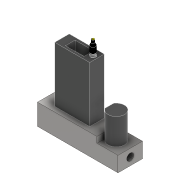
# Autodesk Inventor part: alicat_flujo
Saved by Autodesk Inventor 2022 (Build 260153000, 153)
## iProperties
Created: 2022-11-15
Part Number: alicat_flujo
Material: Generic
Document SubType Name: Modeling
Designer: ferna
Density: 1 g/cm^3
Appearance: Default
Author: ferna
Autodesk Inventor part; units mm, degrees
ref_plane "YZ Plane" through (0, 0, 0) normal (1, 0, 0) x (0, 1, 0)
ref_plane "XZ Plane" through (0, 0, 0) normal (0, 1, 0) x (-1, 0, 0)
sketch "Sketch1" plane through (0, 0, 0) normal (0, 1, 0) x (-1, 0, 0)
  line L0 (0, 0) -> (138, 0)
  line L1 (138, 0) -> (138, -42)
  line L2 (138, -42) -> (0, -42)
  line L3 (0, -42) -> (0, 0)
  dimension "d0" = 138
  dimension "d1" = 42
  constraints: 8 end point, 2 parallel, 1 horizontal, 1 perpendicular
  measures "d0" distance of L1.end L2.end
  measures "d1" distance of L0.end L1.end
extrude "Extrusion1" add sketch "Sketch1" along normal blind 26
sketch "Sketch2" plane through (0, 26, 0) normal (0, 1, 0) x (1, 0, 0)
  line L0 (-138, 42) -> (-138, 0) projected
  line L1 (0, 42) -> (-138, 42) projected
  line L2 (-138, 0) -> (-36, 0)
  line L3 (-36, 0) -> (-36, 42)
  line L4 (-36, 42) -> (-138, 42)
  line L5 (-138, 42) -> (-138, 0)
  point P0 (0, 0)
  dimension "d4" = 102
  constraints: 8 end point, 2 parallel, 1 horizontal, 1 perpendicular, 1 point on line
  measures "d4" distance of L4.end L3.end
extrude "Extrusion2" add sketch "Sketch2" along normal blind 10
sketch "Sketch3" plane through (0, 26, 0) normal (0, 1, 0) x (1, 0, 0)
  line L0 (-36, 0) -> (-36, 42) projected
  line L1 (-36, 21) -> (-24, 21)
  arc A0 (-36, 13.7889) -> (-36, 28.2111) centre (-24, 21) ccw
  line L2 (-36, 13.7889) -> (-36, 28.2111)
  point P0 (0, 0)
  dimension "d7" = 12
  dimension "d8" = 14
  constraints: 4 end point, 2 point on circle, 1 centre point, 1 coincident, 1 collinear, 1 horizontal, 1 midpoint, 1 point on line
  measures "d7" distance of L1.start L1.end
  measures "d8" radius of A0
extrude "Extrusion3" add sketch "Sketch3" along normal blind 45
sketch "Sketch4" plane through (0, 36, 0) normal (0, 1, 0) x (1, 0, 0)
  line L0 (-138, 42) -> (-138, 0) projected
  line L1 (-138, 0) -> (-87, 0)
  line L2 (-138, 0) -> (-36, 0) projected
  line L3 (-87, 0) -> (-87, 21)
  line L4 (-36, 42) -> (-138, 42) projected
  line L5 (-57, 8.5) -> (-117, 8.5)
  line L6 (-117, 8.5) -> (-117, 33.5)
  line L7 (-117, 33.5) -> (-57, 33.5)
  line L8 (-57, 33.5) -> (-57, 8.5)
  line L9 (-57, 8.5) -> (-117, 33.5) construction
  line L10 (-117, 8.5) -> (-57, 33.5) construction
  point P0 (0, 0)
  dimension "d11" = 21
  dimension "d12" = 60
  dimension "d13" = 25
  constraints: 16 end point, 3 midpoint, 2 parallel, 2 perpendicular, 1 horizontal
  measures "d11" distance of L1.end L3.end
  measures "d12" distance of L6.end L7.end
  measures "d13" distance of L5.end L6.end
extrude "Extrusion4" add sketch "Sketch4" along normal blind 95
sketch "Sketch6" plane through (-138, 0, 0) normal (0, 0, 1) x (1, 0, 0)
  line L0 (138, 26) -> (102, 26) projected
  line L1 (102, 26) -> (138, 26)
  line L2 (138, 26) -> (138, 79.7239)
  line L3 (138, 79.7239) -> (98.9473, 78.614)
  line L4 (102, 26) -> (102, 36) projected
  line L5 (98.9473, 78.614) -> (102, 36)
  line L6 (102, 36) -> (102, 26)
  point P0 (138, 0)
  constraints: 10 end point, 2 collinear, 1 perpendicular
split body "Split1" sketch "Sketch6" result two bodies curves L2 L3 L5 L6 L1 first body at (-23.4126, 56, -34.4872)
sketch "Sketch7" plane through (-138, 0, 0) normal (0, 0, 1) x (1, 0, 0)
  line L0 (81, 36) -> (21, 36) projected
  line L1 (81, 36) -> (81, 131) projected
  line L2 (21, 131) -> (81, 131) projected
  line L3 (21, 36) -> (21, 131) projected
  point P0 (138, 0)
split body "Split2" sketch "Sketch7" result two bodies bodies 3 curves L1 L2 L3 L0 first body at (-97, 67.6667, -9)
sketch "Sketch8" plane through (0, 0, 0) normal (1, 0, 0) x (0, 0, -1)
  line L0 (0, 0) -> (42, 0) projected
  line L1 (21, 0) -> (21, 13)
  circle A0 centre (21, 13) radius 6
  dimension "d16" = 13
  dimension "d17" = 12
  constraints: 2 end point, 1 centre point, 1 coincident, 1 midpoint, 1 vertical
  measures "d16" distance of L1.start L1.end
  measures "d17" diameter of A0
extrude "Extrusion5" cut sketch "Sketch8" against normal blind 20 bodies 5
sketch "Sketch9" plane through (-138, 0, -42) normal (-1, 0, 0) x (0, 0, 1)
  circle A0 centre (21, 13) radius 6 projected
  point P0 (42, 0)
extrude "Extrusion6" cut sketch "Sketch9" against normal blind 20 bodies 5
thread "Thread1" size "M12x1.75" class "6H" standard "ANSI Metric M Profile" full length
sketch "Sketch12" plane through (-57, 131, -33.5) normal (0, 0, -1) x (-1, 0, 0)
  line L0 (0.306, -7.7857) -> (59.5727, -7.7857) construction
  line L1 (59.5727, -7.7857) -> (59.5727, -94.7807) construction
  line L2 (59.5727, -94.7807) -> (0.306, -94.7807) construction
  line L3 (0.306, -94.7807) -> (0.306, -7.7857) construction
  point P0 (-57, -131)
  constraints: 2 other
decal "Decal2"
sketch "Sketch13" plane through (0, 131, 0) normal (0, 1, 0) x (1, 0, 0)
  line L0 (-117, 33.5) -> (-117, 8.5) projected
  line L1 (-117, 21) -> (-87, 21)
  line L2 (-102.9, 29.325) -> (-71.1, 29.325)
  line L3 (-71.1, 29.325) -> (-71.1, 12.675)
  line L4 (-71.1, 12.675) -> (-102.9, 12.675)
  line L5 (-102.9, 12.675) -> (-102.9, 29.325)
  line L6 (-102.9, 29.325) -> (-71.1, 12.675) construction
  line L7 (-71.1, 29.325) -> (-102.9, 12.675) construction
  point P0 (0, 0)
  dimension "d38" = 30
  dimension "d39" = 31.8
  dimension "d40" = 16.65
  constraints: 14 end point, 3 midpoint, 2 horizontal, 2 parallel, 1 perpendicular
  measures "d38" distance of L1.start L1.end
  measures "d39" distance of L3.end L4.end
  measures "d40" distance of L2.end L3.end
extrude "Extrusion7" cut sketch "Sketch13" against normal blind 16.2 bodies 4
sketch "Sketch14" plane through (0, 131, 0) normal (0, 1, 0) x (1, 0, 0)
  line L0 (-71.1, 29.325) -> (-71.1, 12.675) projected
  line L1 (-71.1, 21) -> (-63.898, 21)
  circle A0 centre (-63.898, 21) radius 4
  point P0 (0, 0)
  dimension "d52" = 7.202
  dimension "d53" = 8
  constraints: 2 end point, 1 centre point, 1 coincident, 1 horizontal, 1 midpoint
  measures "d52" distance of L1.start L1.end
  measures "d53" diameter of A0
extrude "Extrusion8" add sketch "Sketch14" along normal blind 6 separate body
thread "Thread2" size "M8x1.25" class "6g" standard "ANSI Metric M Profile" full length
sketch "Sketch16" plane through (0, 131, 0) normal (0, 1, 0) x (1, 0, 0)
  circle A0 centre (-63.898, 21) radius 3 projected
  circle A1 centre (-63.898, 21) radius 4 projected
  line L0 (-63.4389, 15.8287) -> (-68.1469, 18.0167)
  line L1 (-68.1469, 18.0167) -> (-68.606, 23.188)
  line L2 (-68.606, 23.188) -> (-64.3571, 26.1713)
  line L3 (-64.3571, 26.1713) -> (-59.6491, 23.9833)
  line L4 (-59.6491, 23.9833) -> (-59.19, 18.812)
  line L5 (-59.19, 18.812) -> (-63.4389, 15.8287)
  point P0 (0, 0)
  constraints: 12 end point, 1 coincident, 13 other
extrude "Extrusion10" add sketch "Sketch16" along normal blind 2 separate body contours A0 | A1 | L0 L1 L2 L3 L4 L5
sketch "Sketch17" plane through (-63.898, 137, -21) normal (0, 1, 0) x (1, 0, 0)
  circle A0 centre (0, 0) radius 3
  point P0 (63.898, -21)
  dimension "d63" = 6
  constraints: 1 centre point
  measures "d63" diameter of A0
extrude "Extrusion11" cut sketch "Sketch17" against normal blind 6 bodies 6 7
sketch "Sketch18" plane through (-63.898, 137, -21) normal (0, 1, 0) x (1, 0, 0)
  circle A0 centre (0, 0) radius 4.5
  point P0 (63.898, -21)
  dimension "d66" = 9
  constraints: 1 centre point
  measures "d66" diameter of A0
extrude "Extrusion12" add sketch "Sketch18" along normal blind 10 separate body
ref_plane "Work Plane1" through (-63.898, 151, -21) normal (0, 1, 0) x (1, 0, 0)
sketch "Sketch19" plane through (-63.898, 151, -21) normal (0, 1, 0) x (1, 0, 0)
  circle A0 centre (0, 0) radius 2.5
  point P0 (63.898, -21)
  dimension "d70" = 5
  constraints: 1 centre point
  measures "d70" diameter of A0
extrude "Extrusion13" add sketch "Sketch19" along normal blind 5 separate body
loft "Loft1" add bodies 8 section 1 edges at (-68.398, 147, -21) section 2 edges at (-66.398, 151, -21)
combine bodies "Combine1" operation type add bodies to combine 9 8
sketch "Sketch20" plane through (-63.898, 156, -21) normal (0, 1, 0) x (1, 0, 0)
  circle A0 centre (0, 0) radius 2.5 projected
body "Solid6"
body "Solid7"
body "Solid8"
body "Solid2"
body "Solid4"
body "Solid5"
